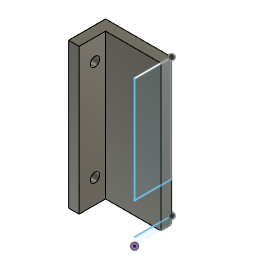
Sensors mounting (Autodesk Fusion 360 design; units mm, degrees)
Autodesk Fusion 360 part; units mm, degrees
sketch "Szkic3" plane through (0, 0, 0) normal (0, 0, 1) x (1, 0, 0)
  line L0 (0, 0) -> (4, 0)
  line L1 (4, 0) -> (4, 10)
  line L2 (4, 10) -> (25, 10)
  line L3 (25, 10) -> (25, 14)
  line L4 (25, 14) -> (0, 14)
  line L5 (0, 14) -> (0, 0)
  constraint coincident L0.start L5.end
  constraint horizontal L0
  constraint perpendicular L0 L1
  constraint perpendicular L1 L2
  constraint perpendicular L2 L3
  constraint perpendicular L3 L4
  constraint perpendicular L0 L5
extrude "Wyciągnięcie proste3" add sketch "Szkic3" along normal blind 55
sketch "Szkic4" plane through (4, 0, 0) normal (1, 0, 0) x (0, 1, 0)
  line L0 (0, 0) -> (10, 0)
  line L1 (10, 0) -> (10, 55)
  line L2 (10, 55) -> (0, 55)
  line L3 (0, 55) -> (0, 0)
  circle A0 centre (6, 9) radius 1.75
  circle A1 centre (6, 47) radius 1.75
  dimension "d19" = 38
  dimension "d20" = 3.5
  dimension "d21" = 3.5
  measures "d19" distance of A0.centre A1.centre
  measures "d20" diameter of A0
  measures "d21" diameter of A1
extrude "Wyciągnięcie proste4" cut sketch "Szkic4" against normal blind 4 contours A0 | A1
sketch "Szkic5" plane through (25, 0, 0) normal (1, 0, 0) x (0, 1, 0)
  line L0 (10, 0) -> (14, 0)
  line L1 (14, 0) -> (14, 55)
  line L2 (14, 55) -> (10, 55)
  line L3 (10, 55) -> (10, 0)
  line L4 (14, 55) -> (0, 55)
  line L5 (0, 55) -> (0, 15)
  line L6 (0, 15) -> (14, 15)
  line L7 (14, 15) -> (14, 55)
  line L8 (14, 3) -> (0, 3)
  line L9 (0, 3) -> (0, 0)
  line L10 (0, 0) -> (14, 0)
  line L11 (14, 0) -> (14, 3)
  constraint horizontal L4
  constraint vertical L5
  constraint horizontal L6
  constraint vertical L7
  constraint coincident L1.end L2.start
  constraint horizontal L8
  constraint vertical L9
  constraint horizontal L10
  constraint vertical L11
  constraint coincident L9.end L10.start
  constraint coincident L1 L8.start
sketch "Szkic6" plane through (0, 14, 0) normal (0, 1, 0) x (-1, 0, 0)
  line L0 (-25, 0) -> (0, 0)
  line L1 (0, 0) -> (0, 55)
  line L2 (0, 55) -> (-25, 55)
  line L3 (-25, 55) -> (-25, 0)
  line L4 (-10, 49) -> (-4, 49)
  line L5 (-4, 49) -> (-4, 29)
  line L6 (-4, 29) -> (-10, 29)
  circle A0 centre (-7, 45) radius 1.8
  line L7 (-5, 20) -> (-15, 20)
  line L8 (-15, 20) -> (-15, 6)
  line L9 (-15, 6) -> (-5, 6)
  line L10 (-5, 6) -> (-5, 20)
  line L11 (-10, 29) -> (-14, 29)
  line L12 (-14, 29) -> (-14, 49)
  line L13 (-14, 49) -> (-10, 49)
  circle A1 centre (-7, 33) radius 1.8
  dimension "d24" = 3.6
  dimension "d25" = 10
  dimension "d26" = 14
  dimension "d27" = 3.6
  constraint horizontal L4
  constraint vertical L5
  constraint horizontal L6
  constraint horizontal L7
  constraint vertical L8
  constraint horizontal L9
  constraint vertical L10
  constraint horizontal L11
  constraint vertical L12
  constraint horizontal L13
  measures "d24" diameter of A0
  measures "d25" distance of L7.start L7.end
  measures "d26" distance of L7.start L9.end
  measures "d27" diameter of A1
extrude "Wyciągnięcie proste5" add sketch "Szkic6" along normal blind 6 contours L4 L5 L6 L11 L12 L13 | L7 L8 L9 L10
